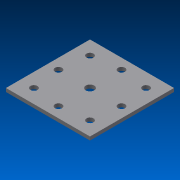
# Autodesk Inventor part: CouplerBridge
Saved by Autodesk Inventor 2013 (Build 170138000, 138)
## iProperties
Created: 2013-07-18
Part Number: CouplerBridge
Material: Generic
Document SubType Name: Modeling
Designer: root
Density: 1 g/cm^3
Author: root
Autodesk Inventor part; units mm, degrees
ref_plane "YZ Plane" through (0, 0, 0) normal (1, 0, 0) x (0, 1, 0)
ref_plane "XZ Plane" through (0, 0, 0) normal (0, 1, 0) x (-1, 0, 0)
ref_plane "XY Plane" through (0, 0, 0) normal (0, 0, 1) x (1, 0, 0)
sketch "Sketch1" plane through (0, 0, 0) normal (0, 1, 0) x (-1, 0, 0)
  line L0 (0, 0) -> (-76.2, 0)
  line L1 (-76.2, 0) -> (-76.2, -76.2)
  line L2 (-76.2, -76.2) -> (0, -76.2)
  line L3 (0, -76.2) -> (0, 0)
  dimension "d0" = 76.2
  dimension "d1" = 76.2
  constraints: 8 end point, 2 parallel, 1 horizontal, 1 perpendicular
  measures "d0" distance of L2.end L0.start
  measures "d1" distance of L1.end L2.end
extrude "Extrusion1" add sketch "Sketch1" along normal blind 3.175
sketch "Sketch2" plane through (0, 3.175, 0) normal (0, 1, 0) x (1, 0, 0)
  line L0 (76.2, 76.2) -> (0, 76.2) projected
  line L1 (0, 76.2) -> (0, 0) projected
  line L2 (9.525, 38.1) -> (38.1, 66.675)
  line L3 (38.1, 66.675) -> (66.675, 38.1)
  line L4 (66.675, 38.1) -> (38.1, 9.525)
  line L5 (38.1, 9.525) -> (9.525, 38.1)
  line L6 (0, 0) -> (76.2, 0) projected
  dimension "d5" = 57.15
  dimension "d7" = 57.15
  dimension "d8" = 9.525
  dimension "d9" = 9.525
  dimension "d29" = 45
  constraints: 8 end point, 4 coincident, 2 parallel, 1 perpendicular
  measures "d5" distance of L2.start L3.end
  measures "d7" distance of L4.end L2.end
  measures "d8" distance from line of L2.end L0
  measures "d9" distance from line of L1 L2.start
  measures "d29" angle of L6 L5
hole "Hole1" at (38.1, 3.175, -66.675) at (9.525, 3.175, -38.1) at (38.1, 3.175, -9.525) at (66.675, 3.175, -38.1) direction (0, -1, 0) diameter 6.35 end through all
sketch "Sketch3" plane through (0, 3.175, 0) normal (0, 1, 0) x (1, 0, 0)
  line L0 (76.2, 0) -> (76.2, 76.2) projected
  line L1 (76.2, 76.2) -> (0, 76.2) projected
  line L2 (12.7, 63.5) -> (63.5, 63.5)
  line L3 (63.5, 63.5) -> (63.5, 12.7)
  line L4 (63.5, 12.7) -> (12.7, 12.7)
  line L5 (12.7, 12.7) -> (12.7, 63.5)
  dimension "d17" = 50.8
  dimension "d19" = 50.8
  dimension "d20" = 12.7
  dimension "d21" = 12.7
  constraints: 8 end point, 4 coincident, 2 parallel, 1 horizontal, 1 perpendicular
  measures "d17" distance of L4.end L2.start
  measures "d19" distance of L3.end L4.end
  measures "d20" distance between parallel lines of L2 L1
  measures "d21" distance between parallel lines of L0 L3
hole "Hole2" at (12.7, 3.175, -63.5) at (63.5, 3.175, -63.5) at (12.7, 3.175, -12.7) at (63.5, 3.175, -12.7) direction (0, -1, 0) diameter 6.35 end through all
sketch "Sketch4" plane through (0, 3.175, 0) normal (0, 1, 0) x (1, 0, 0)
  line L0 (0, 0) -> (76.2, 0) projected
  line L1 (76.2, 0) -> (76.2, 76.2) projected
  point P0 (38.1, 38.1)
  dimension "d34" = 38.1
  dimension "d35" = 38.1
  measures "d34" distance from line of L1 point (38.1, 38.1)
  measures "d35" distance from line of L0 point (38.1, 38.1)
hole "Hole3" at (38.1, 3.175, -38.1) direction (0, -1, 0) diameter 7.62 end through all
body "Solid1"
